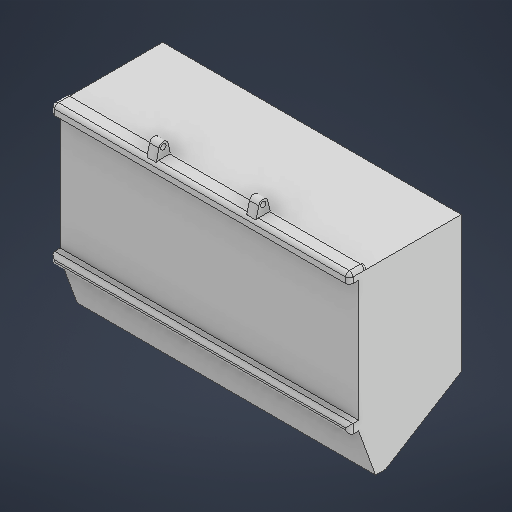
# Autodesk Inventor part: plate2
Saved by Autodesk Inventor 2027 (Build 310192000, 192)
## iProperties
Created: 2026-07-09
Part Number: plate2
Material: Generic
Document SubType Name: Modeling
Designer: uchiha
Density: 1 g/cm^3
Appearance: Default
Author: uchiha
Autodesk Inventor part; units mm, degrees
sketch "Sketch1" plane through (0, 0, 0) normal (0, 0, 1) x (1, 0, 0)
  line L0 (40, 37.5) -> (-40, 37.5)
  line L1 (-40, 37.5) -> (-40, -37.5)
  line L2 (-40, -37.5) -> (40, -37.5)
  line L3 (40, -37.5) -> (40, 37.5)
  line L4 (40, 37.5) -> (-40, -37.5) construction
  line L5 (-40, 37.5) -> (40, -37.5) construction
  point P0 (0, 0)
  dimension "d0" = 80
  dimension "d1" = 75
  constraints: 12 end point, 2 midpoint, 2 parallel, 1 horizontal, 1 perpendicular
  measures "d0" distance of L0.start L0.end
  measures "d1" distance of L2.end L0.start
extrude "Extrusion1" add sketch "Sketch1" along normal blind 10
ref_plane "Work Plane1" through (-13.25, -37.5, 0) normal (1, 0, 0) x (0, 0, -1)
sketch "Sketch2" plane through (-13.25, -37.5, 0) normal (1, 0, 0) x (0, 0, -1)
  circle A0 centre (-5.3658, 80) radius 2.5
  line L0 (0, 75) -> (-10, 75) projected
  line L1 (-9.1092, 75) -> (-7.7995, 80.572)
  line L2 (-2.9321, 80.572) -> (-1.6224, 75)
  point P0 (0, 37.5)
  dimension "d5" = 5
  dimension "d11" = 5
  constraints: 4 end point, 2 point on circle, 2 point on line, 2 tangent, 1 centre point, 1 equal length
  measures "d5" diameter of A0
  measures "d11" distance from line of L0 A0.centre
extrude "Extrusion2" add sketch "Sketch2" along normal mid plane 5
sketch "Sketch3" plane through (-10.75, -37.5, 0) normal (1, 0, 0) x (0, 0, -1)
  arc A0 (-2.9321, 80.572) -> (-7.7995, 80.572) centre (-5.3658, 80) ccw projected
  circle A1 centre (-5.3658, 80) radius 1.5
  point P0 (0, 37.5)
  dimension "d8" = 3
  constraints: 1 centre point, 1 coincident
  measures "d8" diameter of A1
extrude "Extrusion3" cut sketch "Sketch3" against normal blind 20
sketch "Sketch4" plane through (0, 0, 0) normal (0, 0, -1) x (-1, 0, 0)
  point P0 (0, 0)
sketch "Sketch5" plane through (-40, -37.5, 0) normal (-1, 0, 0) x (0, 0, 1)
  point P0 (0, 37.5)
ref_plane "Work Plane2" through (-40, -37.5, 0) normal (-1, 0, 0) x (0, 0, 1)
mirror "Mirror1" about plane through (-40, 37.5, 0) normal (-1, 0, 0) of "Extrusion2", "Extrusion1"
fillet "Fillet1" radius 2 2 edges at (-40, 37.5, 10) (-40, 37.5, 0)
sketch "Sketch6" plane through (-69.25, 42.5, 5.3658) normal (-1, 0, 0) x (0, 0, 1)
  circle A0 centre (0, 0) radius 1.5
  point P0 (-5.3658, -42.5)
  constraints: 1 centre point
extrude "Extrusion4" cut sketch "Sketch6" against normal blind 20
ref_plane "Work Plane3" through (20, 35.5, 6) normal (0, 0, -1) x (-1, 0, 0)
sketch "Sketch7" plane through (40, -37.5, 0) normal (0, -1, 0) x (1, 0, 0)
  line L0 (-160, 8) -> (-160, 10) projected
  line L1 (0, 2) -> (0, 8) projected
  line L2 (-160, 10) -> (0, 10)
  line L3 (0, 10) -> (0, 5)
  line L4 (0, 5) -> (-160, 5)
  line L5 (-160, 5) -> (-160, 10)
  point P0 (-40, 0)
  constraints: 8 end point, 2 parallel, 1 horizontal, 1 midpoint, 1 perpendicular
extrude "Extrusion5" cut sketch "Sketch7" against normal blind 70
fillet "Fillet2" radius 2 14 edges at (-40, -37.5, 5) (-40, -37.5, 0) (40, -2.5, 5) (40, 36.9142, 0.5858) (40, 37.5, 5) (40, 36.9142, 9.4142) (40, 34, 10) (40, -1, 0) (-120, -2.5, 5) (-120, 36.9142, 0.5858) (-120, 37.5, 5) (-120, 36.9142, 9.4142) (-120, 34, 10) (-120, -1, 0)
sketch "Sketch8" plane through (-118, -35.5, 5) normal (0, 0, 1) x (1, 0, 0)
  line L0 (-2, -2) -> (158, -2) projected
  line L1 (156, 73) -> (107.25, 73) projected
  line L2 (158, -2) -> (150.679, -2)
  line L3 (150.679, -2) -> (150.679, 73)
  line L4 (150.679, 73) -> (158, 73)
  line L5 (158, 73) -> (158, -2)
  line L6 (0, 0) -> (-2, -2) projected
  line L7 (0, 68) -> (156, 68) projected
  line L8 (-2, -2) -> (3.321, -2)
  line L9 (3.321, -2) -> (3.321, 68)
  line L10 (3.321, 68) -> (-2, 68)
  line L11 (-2, 68) -> (-2, -2)
  line L12 (-2, 68) -> (158, 68)
  line L13 (158, 68) -> (158, 73)
  line L14 (158, 73) -> (-2, 73)
  line L15 (-2, 73) -> (-2, 68)
  line L16 (156, 68) -> (156, 0) projected
  point P0 (118, 35.5)
  point P1 (156, 34)
  point P2 (150.679, 68)
  point P3 (150.679, -2)
  point P4 (3.321, -2)
  dimension "d19" = 5.321
  dimension "d20" = 5.321
  constraints: 24 end point, 6 parallel, 3 horizontal, 3 perpendicular, 2 point on line, 1 midpoint
  measures "d19" distance from line of point (156, 34) L3
  measures "d20" distance between parallel lines of L11 L9
extrude "Extrusion6" add sketch "Sketch8" against normal blind 55 contours L11 L10 L7 L9 L0 | L3 L7 L12 L5 L0
sketch "Sketch9" plane through (32.679, -37.5, 5) normal (0, -1, 0) x (1, 0, 0)
  point P0 (-32.679, -5)
sketch "Sketch10" plane through (40, -37.5, 5) normal (1, 0, 0) x (0, 0, -1)
  line L0 (0, 2) -> (0, 0) projected
  line L1 (0, 0) -> (18.1985, -50)
  line L2 (18.1985, -50) -> (18.1985, 0)
  line L3 (18.1985, 0) -> (0, 0)
  line L4 (18.1985, -25) -> (9.0993, -25)
  line L5 (13.1985, -21.6436) -> (7.1407, -5)
  line L6 (7.1407, -5) -> (13.1985, -5)
  line L7 (13.1985, -5) -> (13.1985, -21.6436)
  line L8 (7.1407, -5) -> (14.4201, -25)
  line L9 (13.1985, -21.6436) -> (5.3209, 0)
  point P0 (5, 37.5)
  point P1 (9.0993, 0)
  point P2 (7.1407, -5)
  point P3 (13.1985, -21.6436)
  dimension "d23" = 70
  dimension "d24" = 25
  dimension "d25" = 5
  constraints: 18 end point, 4 point on line, 3 midpoint, 2 perpendicular, 1 parallel, 2 other
  measures "d23" angle of L1 L3
  measures "d24" distance from line of L4 point (9.099, 0)
  measures "d25" distance between parallel lines of L1 L5
extrude "Extrusion7" add sketch "Sketch10" against normal up to surface (160 mm away) contours L3 L9 L5 L8 L4 L1
sketch "Sketch11" plane through (40, 35.5, 8) normal (1, 0, 0) x (0, 0, -1)
  line L0 (17.4201, -98) -> (8.3209, -73) projected
  line L1 (58, -73) -> (8.3209, -73) projected
  line L2 (17.4201, -98) -> (58, -73)
  point P0 (8, -35.5)
  constraints: 2 end point
extrude "Extrusion8" add sketch "Sketch11" against normal up to surface (7.321 mm away)
sketch "Sketch12" plane through (-120, 35.5, 2) normal (-1, 0, 0) x (0, 0, 1)
  line L0 (-52, -73) -> (-52, -3) projected
  line L1 (-2.3209, -73) -> (-11.4201, -98) projected
  line L2 (-52, -73) -> (-11.4201, -98)
  line L3 (-2.3209, -73) -> (-52, -73)
  point P0 (-2, -35.5)
  constraints: 4 end point, 1 perpendicular
extrude "Extrusion9" add sketch "Sketch12" against normal up to surface (5.321 mm away)
sketch "Sketch13" plane through (-118, -35.5, -50) normal (0, 0, -1) x (-1, 0, 0)
  point P0 (-118, 35.5)
sketch "Sketch14" plane through (32.679, -35.5, 0) normal (-1, 0, 0) x (0, 0, 1)
  point P0 (0, 35.5)
sketch "Sketch15" plane through (-120, -62.5, -9.4201) normal (0, -0.851398, -0.5245201) x (1, 0, 0)
  point P0 (120, -24.7622)
ref_plane "Work Plane4" through (-120, 32.5, 5) normal (0.7071068, 0, 0.7071068) x (0, 1, 0)
sketch "Sketch16" plane through (-120, 32.5, 5) normal (0, 0, 1) x (1, 0, 0)
  line L0 (152.679, -68) -> (5.321, -68) projected
  line L1 (152.679, -70) -> (5.321, -70) projected
  line L2 (152.679, -68) -> (152.679, -70) projected
  line L3 (5.321, -70) -> (5.321, -68) projected
  point P0 (120, -32.5)
extrude "Extrusion10" add sketch "Sketch16" along normal up to surface surface through (40, -37.5, -0.3209) normal (0, 0.3420201, -0.9396926)
sketch "Sketch17" plane through (0, 0, 0) normal (0, 0, -1) x (-1, 0, 0)
  line L0 (-32.679, -36.2344) -> (114.679, -36.2344) projected
  line L1 (114.679, -35.5) -> (-32.679, -35.5) projected
  line L2 (-32.679, -37.5) -> (-32.679, 32.5) projected
  line L3 (114.679, 32.5) -> (114.679, -37.5) projected
  point P0 (0, 0)
extrude "Extrusion11" add sketch "Sketch17" against normal up to surface surface through (40, -37.5, -0.3209) normal (0, 0.3420201, -0.9396926)
sketch "Sketch18" plane through (0, 0, 0) normal (0, 0, -1) x (-1, 0, 0)
  point P0 (0, 0)
ref_plane "Work Plane5" through (32.679, -62.5, -9.4201) normal (0, 0.3420201, -0.9396926) x (-1, 0, 0)
sketch "Sketch19" plane through (32.679, -62.5, -9.4201) normal (0, 0.3420201, -0.9396926) x (-1, 0, 0)
  line L0 (147.358, 0) -> (147.358, 27.9512) projected
  line L1 (0, 27.9512) -> (147.358, 27.9512) projected
  line L2 (0, 0) -> (0, 27.9512) projected
  line L3 (0, 0) -> (147.358, 0) projected
  point P0 (32.679, 61.9527)
extrude "Extrusion13" add sketch "Sketch19" along normal blind 0.14
sketch "Sketch20" plane through (0, 0, 10) normal (0, 0, 1) x (1, 0, 0)
  line L0 (-114.679, -37.5) -> (-120, -37.5) projected
  line L1 (40, -37.5) -> (40, 32.5) projected
  line L2 (-120, -37.5) -> (40, -37.5)
  line L3 (40, -37.5) -> (40, -32.5)
  line L4 (40, -32.5) -> (-120, -32.5)
  line L5 (-120, -32.5) -> (-120, -37.5)
  line L6 (-118, 32.5) -> (38, 32.5) projected
  line L7 (-15.75, 37.5) -> (-64.25, 37.5) projected
  point P0 (0, 0)
  dimension "d41" = 5
  dimension "d42" = 5
  constraints: 8 end point, 2 parallel, 1 horizontal, 1 perpendicular, 1 point on line
  measures "d41" distance between parallel lines of L6 L7
  measures "d42" distance between parallel lines of L2 L4
extrude "Extrusion14" add sketch "Sketch20" against normal up to surface (5 mm away)
fillet "Fillet3" radius 2 4 edges at (-40, -37.5, 10) (-40, -32.5, 10) (40, -35, 10) (-120, -35, 10)
sketch "Sketch21" plane through (-118, -35.5, -50) normal (0, 0, -1) x (-1, 0, 0)
  line L0 (2, -2) -> (2, 68) projected
  line L1 (-158, 71) -> (2, 71)
  line L2 (2, 71) -> (2, 66)
  line L3 (2, 66) -> (-158, 66)
  line L4 (-158, 66) -> (-158, 71)
  line L5 (0, 71) -> (2, 71) projected
  line L6 (-158, 71) -> (-158, 68) projected
  point P0 (-118, 35.5)
  point P1 (1, 71)
  point P2 (-158, 69.5)
  dimension "d46" = 5
  constraints: 8 end point, 3 point on line, 2 midpoint, 2 parallel, 1 horizontal, 1 perpendicular
  measures "d46" distance between parallel lines of L3 L1
extrude "Extrusion15" add sketch "Sketch21" against normal up to surface (55 mm away)
equation "\"d42\" = d41"
body "Solid1"
